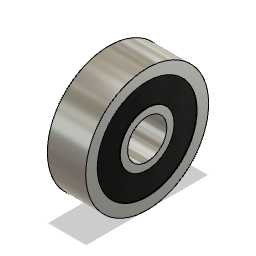
_628 bearing.936f0910-3e04-4f5d-8cef-8d82794ba071 (Autodesk Fusion 360 design; units mm, degrees)
Autodesk Fusion 360 part; units mm, degrees
sketch "Sketch1" plane through (0, 0, 0) normal (1, 0, 0) x (0, 0, -1)
  circle A0 centre (0, 0) radius 2.55
  circle A1 centre (0, 0) radius 8
  circle A2 centre (0, 0) radius 3.5
  circle A3 centre (0, 0) radius 6.5
  dimension "d1" = 5.1
  dimension "d2" = 16
  dimension "d3" = 7
  dimension "d4" = 13
  constraint coincident A0.centre A1.centre
  constraint concentric A0 A1
  constraint concentric A1 A2
  constraint concentric A2 A3
  measures "d1" diameter of A0
  measures "d2" diameter of A1
  measures "d3" diameter of A2
  measures "d4" diameter of A3
extrude "Extrude1" add sketch "Sketch1" along normal blind 5 makes body 1 at (3.3333, -0.3988, -7.9901) makes body 2 at (3.3333, -0.1745, -3.4956)
extrude "Extrude2" add sketch "Sketch1" along normal blind 4.8 from surface at 0.1 separate body contours A3 makes body 3
